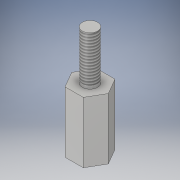
# Autodesk Inventor part: Espacador_Placas
Saved by Autodesk Inventor 2019 (Build 230136000, 136)
## iProperties
Created: 2020-03-13
Part Number: Espacador_Placas
Material: Alumínio 6061
Document SubType Name: Modeling
Designer: caio.santos
Density: 2.7 g/cm^3
Appearance: Alumínio - Polido
Author: caio.santos
Autodesk Inventor part; units mm, degrees
ref_plane "YZ Plane" through (0, 0, 0) normal (1, 0, 0) x (0, 1, 0)
ref_plane "XZ Plane" through (0, 0, 0) normal (0, 1, 0) x (-1, 0, 0)
ref_plane "XY Plane" through (0, 0, 0) normal (0, 0, 1) x (1, 0, 0)
sketch "Esboço1" plane through (0, 0, 0) normal (0, 1, 0) x (-1, 0, 0)
  line L0 (-1.5, -2.5981) -> (1.5, -2.5981)
  line L1 (-1.5, 2.5981) -> (1.5, 2.5981)
  line L2 (1.5, 2.5981) -> (3, 0)
  line L3 (1.5, -2.5981) -> (3, 0)
  line L4 (-1.5, 2.5981) -> (-3, 0)
  line L5 (-3, 0) -> (-1.5, -2.5981)
  point P0 (0, 0)
  dimension "d8" = 3
  dimension "d10" = 3
  dimension "d11" = 3
  dimension "d12" = 3
  dimension "d15" = 1.5
  dimension "d16" = 1.5
  dimension "d17" = 120
  dimension "d18" = 120
  dimension "d19" = 120
  dimension "d20" = 120
  dimension "d21" = 120
  dimension "d22" = 2.5981
  constraints: 12 end point
  measures "d8" distance of L0.start L0.end
  measures "d10" distance of L1.start L1.end
  measures "d11" distance of L0.end L2.end
  measures "d12" distance of L1.end L2.end
  measures "d15" horizontal distance of point (0, 0) L1.start
  measures "d16" horizontal distance of L0.start point (0, 0)
  measures "d17" angle of L3 L2
  measures "d18" angle of L1 L2
  measures "d19" angle of L0 L3
  measures "d20" angle of L1 L4
  measures "d21" angle of L5 L0
  measures "d22" distance from line of point (0, 0) L2
extrude "Extrusão1" add sketch "Esboço1" along normal blind 10
sketch "Esboço2" plane through (0, 10, 0) normal (0, 1, 0) x (1, 0, 0)
  circle A0 centre (0, 0) radius 1.25
  dimension "d26" = 2.5
  constraints: 1 centre point, 1 coincident
  measures "d26" diameter of A0
extrude "Extrusão2" add sketch "Esboço2" along normal blind 8
thread "Rosca1" size "M2.5x0.45" class "6g" standard "ANSI Metric M Profile" length 7.5
sketch "Esboço3" plane through (0, 0, 0) normal (0, -1, 0) x (1, 0, 0)
  circle A0 centre (0, 0) radius 1.25
  dimension "d33" = 2.5
  constraints: 1 centre point, 1 coincident
  measures "d33" diameter of A0
extrude "Extrusão3" cut sketch "Esboço3" against normal blind 6
thread "Rosca3" size "M2.5x0.45" class "6H" standard "ANSI Metric M Profile" length 4.5
equation "\"d8\" = 2 * d16"
equation "\"d10\" = 2 * d15"
equation "\"d17\" = d18"
equation "\"d19\" = d18"
equation "\"d20\" = d18"
equation "\"d21\" = d18"
